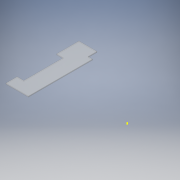
# Autodesk Inventor part: Lexan
Saved by Autodesk Inventor 2016 (Build 200138000, 138)
## iProperties
Created: 2015-11-11
Part Number: Lexan
Material: Acetal Resin, White(1)
Document SubType Name: Modeling
Designer: Julia
Density: 1.425 g/cm^3
Appearance: Smooth - White(1)
Author: Julia
Autodesk Inventor part; units mm, degrees
ref_plane "YZ Plane" through (0, 0, 0) normal (1, 0, 0) x (0, 1, 0)
ref_plane "XZ Plane" through (0, 0, 0) normal (0, 1, 0) x (-1, 0, 0)
ref_plane "XY Plane" through (0, 0, 0) normal (0, 0, 1) x (1, 0, 0)
sketch "Sketch1" plane through (0, 0, 0) normal (0, 1, 0) x (-1, 0, 0)
  line L0 (542.2576, 149.421) -> (414.2963, 149.421)
  line L1 (414.2963, 149.421) -> (414.2963, -266.7891)
  line L2 (414.2963, -266.7891) -> (542.2576, -266.7891)
  line L3 (542.2576, -266.7891) -> (542.2576, 149.421)
  point P0 (0, 0)
  constraints: 8 end point, 2 parallel, 1 horizontal, 1 perpendicular
extrude "Extrusion1" add sketch "Sketch1" along normal blind 4.7498
sketch "Sketch2" plane through (0, 0, 0) normal (0, -1, 0) x (1, 0, 0)
  point P0 (0, 0)
sketch "Sketch3" plane through (0, 0, 0) normal (0, -1, 0) x (1, 0, 0)
  line L0 (-542.2576, 149.421) -> (-414.2963, 149.421) projected
  line L1 (-542.2576, 149.421) -> (-542.2576, 22.421)
  line L2 (-542.2576, -266.7891) -> (-542.2576, 149.421) projected
  line L3 (-414.2963, -266.7891) -> (-542.2576, -266.7891) projected
  line L4 (-542.2576, -266.7891) -> (-542.2576, -139.7891)
  line L5 (-542.2576, -139.7891) -> (-504.1576, -139.7891)
  line L6 (-504.1576, -139.7891) -> (-504.1576, 22.421)
  line L7 (-504.1576, 22.421) -> (-542.2576, 22.421)
  line L8 (-504.1576, -139.7891) -> (-542.2576, -139.7891)
  line L9 (-542.2576, -139.7891) -> (-542.2576, 22.421)
  line L10 (-542.2576, 22.421) -> (-504.1576, 22.421)
  line L11 (-504.1576, 22.421) -> (-504.1576, -139.7891)
  point P0 (0, 0)
  dimension "d2" = 127
  dimension "d3" = 127
  dimension "d4" = 38.1
  constraints: 18 end point, 3 perpendicular, 2 horizontal, 2 parallel, 2 point on line
  measures "d2" distance of L0.start L1.end
  measures "d3" distance of L2.start L4.end
  measures "d4" distance of L4.end L5.end
extrude "Extrusion2" cut sketch "Sketch3" against normal blind 65.0875
sketch "Sketch4" plane through (0, 0, 0) normal (0, -1, 0) x (1, 0, 0)
  point P0 (0, 0)
sketch "Sketch5" plane through (0, 0, 0) normal (0, -1, 0) x (1, 0, 0)
  line L0 (-542.2576, 22.421) -> (-542.2576, 85.921)
  line L1 (-542.2576, 22.421) -> (-542.2576, 149.421) projected
  line L2 (-510.2194, 85.921) -> (-510.2194, 22.421)
  line L3 (-542.2576, 22.421) -> (-504.1576, 22.421) projected
  line L4 (-542.2576, 85.921) -> (-510.2194, 85.921)
  point P0 (0, 0)
  constraints: 6 end point, 1 midpoint, 1 parallel, 1 perpendicular, 1 point on line
sketch "Sketch6" plane through (0, 0, 0) normal (0, -1, 0) x (1, 0, 0)
  point P0 (0, 0)
extrude "Extrusion3" cut sketch "Sketch5" against normal blind 123.825
sketch "Sketch7" plane through (0, 4.7498, 0) normal (0, 1, 0) x (1, 0, 0)
  line L0 (-414.2963, -149.421) -> (-414.2963, 266.7891) projected
  line L1 (-414.2963, 266.7891) -> (-433.3463, 266.7891)
  line L2 (-414.2963, 266.7891) -> (-542.2576, 266.7891) projected
  line L3 (-433.3463, 266.7891) -> (-433.3463, 215.9891)
  line L4 (-433.3463, 215.9891) -> (-414.2963, 215.9891)
  point P0 (0, 0)
  dimension "d9" = 19.05
  dimension "d11" = 50.8
  constraints: 6 end point, 2 perpendicular, 2 point on line
  measures "d9" distance of L0.end L1.end
  measures "d11" distance of L1.end L3.end
extrude "Extrusion4" cut sketch "Sketch7" against normal blind 42.8625
sketch "Sketch8" plane through (0, 4.7498, 0) normal (0, 1, 0) x (1, 0, 0)
  line L0 (-510.2194, -22.421) -> (-504.1207, -22.421)
  line L1 (-504.1207, -22.421) -> (-504.1207, -85.7832)
  line L2 (-510.2194, -85.921) -> (-510.2194, -22.421) projected
  line L3 (-510.2194, -85.7832) -> (-510.2194, -22.421)
  line L4 (-542.2576, -85.921) -> (-510.2194, -85.921) projected
  line L5 (-510.2194, -85.7832) -> (-510.2194, -85.921)
  line L6 (-510.2194, -85.921) -> (-504.1207, -85.921)
  line L7 (-504.1207, -85.921) -> (-504.1207, -85.7832)
  point P0 (0, 0)
  constraints: 12 end point, 3 perpendicular, 1 collinear, 1 horizontal, 1 vertical
extrude "Extrusion5" cut sketch "Sketch8" against normal blind 28.575
sketch "Sketch9" plane through (0, 4.7498, 0) normal (0, 1, 0) x (1, 0, 0)
  point P0 (0, 0)
sketch "Sketch10" plane through (0, 4.7498, 0) normal (0, 1, 0) x (1, 0, 0)
  line L0 (-414.2963, 215.9891) -> (-433.3463, 215.9891) projected
  line L1 (-433.3463, 215.9891) -> (-439.6963, 215.9891)
  line L2 (-439.6963, 215.9891) -> (-439.6963, 266.7891)
  line L3 (-433.3463, 266.7891) -> (-542.2576, 266.7891) projected
  line L4 (-433.3463, 266.7891) -> (-433.3463, 215.9891) projected
  line L5 (-433.3463, 266.7891) -> (-433.3463, 215.9891)
  point P0 (0, 0)
  dimension "d16" = 6.35
  constraints: 6 end point, 1 collinear, 1 horizontal, 1 perpendicular, 1 point on line
  measures "d16" distance of L0.end L1.end
extrude "Extrusion6" cut sketch "Sketch10" against normal blind 36.5125
body "Solid1"
